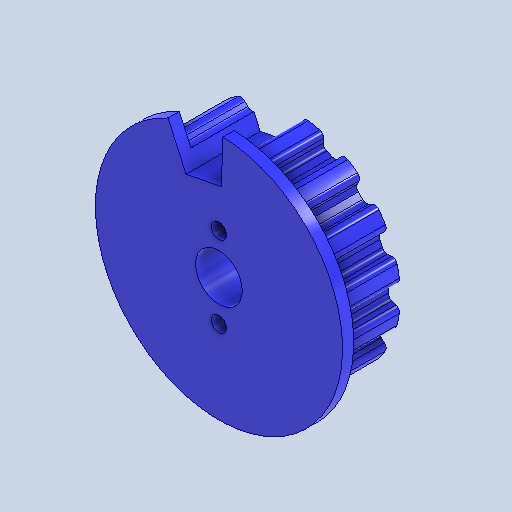
# Autodesk Inventor part: belt_liner_v2_3DP_P-1
Saved by Autodesk Inventor 2025.2 (Build 292293000, 293)
## iProperties
CustomPartVersion: 1
Created: 2024-12-08
Part Number: belt_liner_v2_3DP_P-1
Material: ABS プラスチック
Document SubType Name: Modeling
Designer: haruy
Density: 1.06 g/cm^3
Appearance: 青 - 壁塗料 - 光沢
Author: haruy
Autodesk Inventor part; units mm, degrees
ref_plane "YZ Plane" through (0, 0, 0) normal (1, 0, 0) x (0, 1, 0)
ref_plane "XZ Plane" through (0, 0, 0) normal (0, 1, 0) x (-1, 0, 0)
sketch "プーリ スケッチ" plane through (0, 0, 0) normal (0, 0, 1) x (1, 0, 0)
  circle A0 centre (0, 0) radius 24.2552 construction
  circle A1 centre (0, 0) radius 23.8742
  circle A2 centre (0, 0) radius 21.2072
  line L0 (-2.4489, 23.7483) -> (-1.524, 21.2072)
  line L1 (-1.524, 21.2072) -> (1.524, 21.2072)
  line L2 (1.524, 21.2072) -> (2.4489, 23.7483)
  line L3 (0, 0) -> (0, 23.8742) construction
  point P0 (0, 21.2072)
  dimension "d0" = 48.5104
  dimension "d1" = 0.381
  dimension "d2" = 2.667
  dimension "d3" = 40
  dimension "d4" = 3.048
  constraints: 8 end point, 3 coincident, 3 point on circle, 2 centre point, 1 horizontal, 1 midpoint, 1 point on line, 1 vertical, 1 vertical alignment, 3 other
  measures "d0" diameter of A0
  measures "d1" radial gap between concentric circles of A0 A1
  measures "d3" angle of L2 L0
  measures "d4" distance of L0.end L1.end
extrude "基本ボディ" add sketch "プーリ スケッチ" along normal mid plane 14 contours A2 | A1 L0 L1 L2 | L2 L1 L0 A1
extrude "歯" cut sketch "プーリ スケッチ" along normal through all both and the other way through all contours L2 L1 L0 A1 picked at (0, 22.9759)
fillet "Fillet" radius 1.1938 2 edges at (1.524, 21.2072, 0) (-1.524, 21.2072, 0)
fillet "Fillet" radius 1.1684 4 edges at (-2.4489, 23.7483, 3.5) (-2.4489, 23.7483, -3.5) (2.4489, 23.7483, 3.5) (2.4489, 23.7483, -3.5)
pattern_circular "Teeth" count 16 over 360 about axis through (0, 0, -10) along (0, 0, 1) of "歯", "Fillet"
sketch "スケッチ2" plane through (0, 0, 7) normal (0, 0, 1) x (1, 0, 0)
  circle A0 centre (0, 0) radius 27.5
  dimension "d17" = 55
  constraints: 1 centre point, 1 coincident
  measures "d17" diameter of A0
extrude "押し出し3" add sketch "スケッチ2" along normal blind 2.5
ref_plane "作業平面1" through (0, 0, 0) normal (0, 0, -1) x (-1, 0, 0)
mirror "ミラー1" [suppressed]
sketch "スケッチ3" plane through (0, 0, 9.5) normal (0, 0, 1) x (1, 0, 0)
  circle A0 centre (0, 0) radius 5.2
  circle A1 centre (0, 9) radius 1.7
  circle A2 centre (0, -9) radius 1.7
  dimension "d21" = 10.4
  dimension "d22" = 3.4
  dimension "d23" = 9
  dimension "d26" = 360
  constraints: 3 centre point, 1 coincident, 5 other
  measures "d21" diameter of A0
  measures "d22" diameter of A1
  measures "d23" distance of A1.centre point (0, 0)
extrude "押し出し4" cut sketch "スケッチ3" against normal through all
sketch "スケッチ4" plane through (0, 0, -7) normal (0, 0, -1) x (-1, 0, 0)
  line L0 (-35.8556, 31.439) -> (48.4071, 14.6781)
  arc A0 (5.9069, 23.132) -> (3.395, 23.6316) centre (0, 0) ccw projected
  line L1 (3.395, 23.6316) -> (5.9069, 23.132)
  line L2 (2.199, 23.8695) -> (1.6137, 20.9271)
  line L3 (0, 0) -> (4.6509, 23.3818)
  line L4 (2.6894, 23.772) -> (6.6125, 22.9916)
  line L5 (6.6125, 22.9916) -> (6.0272, 20.0492)
  line L6 (6.0272, 20.0492) -> (2.1041, 20.8296)
  line L7 (2.1041, 20.8296) -> (2.6894, 23.772)
  line L8 (2.199, 23.8695) -> (7.1029, 22.894)
  line L9 (7.1029, 22.894) -> (9.0538, 32.7019)
  line L10 (9.0538, 32.7019) -> (4.1499, 33.6773)
  line L11 (4.1499, 33.6773) -> (2.199, 23.8695)
  line L12 (8.6743, 20.5423) -> (11.4055, 34.2733)
  line L13 (11.4055, 34.2733) -> (2.5785, 36.0291)
  line L14 (2.5785, 36.0291) -> (-0.1528, 22.2981)
  line L15 (1.118, 26.1237) -> (8.9642, 24.563)
  line L16 (8.9642, 24.563) -> (7.5986, 17.6975)
  line L17 (7.5986, 17.6975) -> (-0.2477, 19.2582)
  line L18 (-0.2477, 19.2582) -> (1.118, 26.1237)
  line L19 (-0.1528, 22.2981) -> (-0.7381, 19.3558)
  line L20 (-0.7381, 19.3558) -> (-0.2477, 19.2582)
  line L21 (8.6743, 20.5423) -> (8.089, 17.5999)
  line L22 (8.089, 17.5999) -> (7.5986, 17.6975)
  line L23 (-11.4055, 34.2733) -> (-8.6743, 20.5423)
  line L24 (-8.6743, 20.5423) -> (-8.089, 17.5999)
  line L25 (0.2477, 19.2582) -> (-7.5986, 17.6975)
  line L26 (-8.089, 17.5999) -> (-7.5986, 17.6975)
  line L27 (0.7381, 19.3558) -> (0.2477, 19.2582)
  line L28 (0.1528, 22.2981) -> (0.7381, 19.3558)
  line L29 (0.1528, 22.2981) -> (-2.5785, 36.0291)
  line L30 (-23.6532, 27.2997) -> (-15.8752, 15.6591)
  line L31 (-15.8752, 15.6591) -> (-14.2085, 13.1647)
  line L32 (-7.141, 17.887) -> (-13.7927, 13.4425)
  line L33 (-14.2085, 13.1647) -> (-13.7927, 13.4425)
  line L34 (-6.7252, 18.1648) -> (-7.141, 17.887)
  line L35 (-8.392, 20.6592) -> (-6.7252, 18.1648)
  line L36 (-8.392, 20.6592) -> (-16.1699, 32.2998)
  line L37 (-32.2998, 16.1699) -> (-20.6592, 8.392)
  line L38 (-20.6592, 8.392) -> (-18.1648, 6.7252)
  line L39 (-13.4425, 13.7927) -> (-17.887, 7.141)
  line L40 (-18.1648, 6.7252) -> (-17.887, 7.141)
  line L41 (-13.1647, 14.2085) -> (-13.4425, 13.7927)
  line L42 (-15.6591, 15.8752) -> (-13.1647, 14.2085)
  line L43 (-15.6591, 15.8752) -> (-27.2997, 23.6532)
  line L44 (-36.0291, 2.5785) -> (-22.2981, -0.1528)
  line L45 (-22.2981, -0.1528) -> (-19.3558, -0.7381)
  line L46 (-17.6975, 7.5986) -> (-19.2582, -0.2477)
  line L47 (-19.3558, -0.7381) -> (-19.2582, -0.2477)
  line L48 (-17.5999, 8.089) -> (-17.6975, 7.5986)
  line L49 (-20.5423, 8.6743) -> (-17.5999, 8.089)
  line L50 (-20.5423, 8.6743) -> (-34.2733, 11.4055)
  line L51 (-34.2733, -11.4055) -> (-20.5423, -8.6743)
  line L52 (-20.5423, -8.6743) -> (-17.5999, -8.089)
  line L53 (-19.2582, 0.2477) -> (-17.6975, -7.5986)
  line L54 (-17.5999, -8.089) -> (-17.6975, -7.5986)
  line L55 (-19.3558, 0.7381) -> (-19.2582, 0.2477)
  line L56 (-22.2981, 0.1528) -> (-19.3558, 0.7381)
  line L57 (-22.2981, 0.1528) -> (-36.0291, -2.5785)
  line L58 (-27.2997, -23.6532) -> (-15.6591, -15.8752)
  line L59 (-15.6591, -15.8752) -> (-13.1647, -14.2085)
  line L60 (-17.887, -7.141) -> (-13.4425, -13.7927)
  line L61 (-13.1647, -14.2085) -> (-13.4425, -13.7927)
  line L62 (-18.1648, -6.7252) -> (-17.887, -7.141)
  line L63 (-20.6592, -8.392) -> (-18.1648, -6.7252)
  line L64 (-20.6592, -8.392) -> (-32.2998, -16.1699)
  line L65 (-16.1699, -32.2998) -> (-8.392, -20.6592)
  line L66 (-8.392, -20.6592) -> (-6.7252, -18.1648)
  line L67 (-13.7927, -13.4425) -> (-7.141, -17.887)
  line L68 (-6.7252, -18.1648) -> (-7.141, -17.887)
  line L69 (-14.2085, -13.1647) -> (-13.7927, -13.4425)
  line L70 (-15.8752, -15.6591) -> (-14.2085, -13.1647)
  line L71 (-15.8752, -15.6591) -> (-23.6532, -27.2997)
  line L72 (-2.5785, -36.0291) -> (0.1528, -22.2981)
  line L73 (0.1528, -22.2981) -> (0.7381, -19.3558)
  line L74 (-7.5986, -17.6975) -> (0.2477, -19.2582)
  line L75 (0.7381, -19.3558) -> (0.2477, -19.2582)
  line L76 (-8.089, -17.5999) -> (-7.5986, -17.6975)
  line L77 (-8.6743, -20.5423) -> (-8.089, -17.5999)
  line L78 (-8.6743, -20.5423) -> (-11.4055, -34.2733)
  line L79 (11.4055, -34.2733) -> (8.6743, -20.5423)
  line L80 (8.6743, -20.5423) -> (8.089, -17.5999)
  line L81 (-0.2477, -19.2582) -> (7.5986, -17.6975)
  line L82 (8.089, -17.5999) -> (7.5986, -17.6975)
  line L83 (-0.7381, -19.3558) -> (-0.2477, -19.2582)
  line L84 (-0.1528, -22.2981) -> (-0.7381, -19.3558)
  line L85 (-0.1528, -22.2981) -> (2.5785, -36.0291)
  line L86 (23.6532, -27.2997) -> (15.8752, -15.6591)
  line L87 (15.8752, -15.6591) -> (14.2085, -13.1647)
  line L88 (7.141, -17.887) -> (13.7927, -13.4425)
  line L89 (14.2085, -13.1647) -> (13.7927, -13.4425)
  line L90 (6.7252, -18.1648) -> (7.141, -17.887)
  line L91 (8.392, -20.6592) -> (6.7252, -18.1648)
  line L92 (8.392, -20.6592) -> (16.1699, -32.2998)
  line L93 (32.2998, -16.1699) -> (20.6592, -8.392)
  line L94 (20.6592, -8.392) -> (18.1648, -6.7252)
  line L95 (13.4425, -13.7927) -> (17.887, -7.141)
  line L96 (18.1648, -6.7252) -> (17.887, -7.141)
  line L97 (13.1647, -14.2085) -> (13.4425, -13.7927)
  line L98 (15.6591, -15.8752) -> (13.1647, -14.2085)
  line L99 (15.6591, -15.8752) -> (27.2997, -23.6532)
  line L100 (36.0291, -2.5785) -> (22.2981, 0.1528)
  line L101 (22.2981, 0.1528) -> (19.3558, 0.7381)
  line L102 (17.6975, -7.5986) -> (19.2582, 0.2477)
  line L103 (19.3558, 0.7381) -> (19.2582, 0.2477)
  line L104 (17.5999, -8.089) -> (17.6975, -7.5986)
  line L105 (20.5423, -8.6743) -> (17.5999, -8.089)
  line L106 (20.5423, -8.6743) -> (34.2733, -11.4055)
  line L107 (34.2733, 11.4055) -> (20.5423, 8.6743)
  line L108 (20.5423, 8.6743) -> (17.5999, 8.089)
  line L109 (19.2582, -0.2477) -> (17.6975, 7.5986)
  line L110 (17.5999, 8.089) -> (17.6975, 7.5986)
  line L111 (19.3558, -0.7381) -> (19.2582, -0.2477)
  line L112 (22.2981, -0.1528) -> (19.3558, -0.7381)
  line L113 (22.2981, -0.1528) -> (36.0291, 2.5785)
  line L114 (27.2997, 23.6532) -> (15.6591, 15.8752)
  line L115 (15.6591, 15.8752) -> (13.1647, 14.2085)
  line L116 (17.887, 7.141) -> (13.4425, 13.7927)
  line L117 (13.1647, 14.2085) -> (13.4425, 13.7927)
  line L118 (18.1648, 6.7252) -> (17.887, 7.141)
  line L119 (20.6592, 8.392) -> (18.1648, 6.7252)
  line L120 (20.6592, 8.392) -> (32.2998, 16.1699)
  line L121 (16.1699, 32.2998) -> (8.392, 20.6592)
  line L122 (8.392, 20.6592) -> (6.7252, 18.1648)
  line L123 (13.7927, 13.4425) -> (7.141, 17.887)
  line L124 (6.7252, 18.1648) -> (7.141, 17.887)
  line L125 (14.2085, 13.1647) -> (13.7927, 13.4425)
  line L126 (15.8752, 15.6591) -> (14.2085, 13.1647)
  line L127 (15.8752, 15.6591) -> (23.6532, 27.2997)
  line L128 (13.4918, 31.8191) -> (11.5409, 22.0113)
  line L129 (18.3958, 30.8437) -> (13.4918, 31.8191)
  line L130 (16.4449, 21.0358) -> (18.3958, 30.8437)
  line L131 (11.5409, 22.0113) -> (16.4449, 21.0358)
  line L132 (11.4461, 18.9714) -> (12.0313, 21.9137)
  line L133 (15.3692, 18.191) -> (11.4461, 18.9714)
  line L134 (15.9545, 21.1334) -> (15.3692, 18.191)
  line L135 (22.8338, 29.9609) -> (20.8829, 20.153)
  line L136 (27.7377, 28.9854) -> (22.8338, 29.9609)
  line L137 (25.7868, 19.1776) -> (27.7377, 28.9854)
  line L138 (20.8829, 20.153) -> (25.7868, 19.1776)
  line L139 (20.788, 17.1131) -> (21.3733, 20.0555)
  line L140 (24.7112, 16.3328) -> (20.788, 17.1131)
  line L141 (25.2965, 19.2751) -> (24.7112, 16.3328)
  circle A1 centre (0, 0) radius 27.5
  line L142 (-0.8791, 27.4859) -> (0.7989, 19.05)
  line L143 (11.3306, 25.0573) -> (6.5521, 17.9057)
  line L144 (0.1425, 21.2198) -> (7.9888, 19.6591)
  line L145 (7.9888, 19.6591) -> (7.306, 16.2263)
  line L146 (7.306, 16.2263) -> (-0.5403, 17.787)
  line L147 (-0.5403, 17.787) -> (0.1425, 21.2198)
  line L148 (-0.5403, 17.787) -> (-0.8791, 27.4859)
  line L149 (7.306, 16.2263) -> (11.3306, 25.0573)
  point P0 (4.6576, 23.4155)
  point P1 (0.7187, 19.4532)
  point P2 (7.2808, 18.9963)
  point P3 (11.3306, 25.0573)
  point P4 (11.3306, 25.0573)
  point P5 (7.4069, 17.7356)
  point P6 (-0.056, 19.2201)
  point P7 (0.543, 20.3365)
  point P8 (8.1012, 20.2241)
  point P9 (7.3509, 17.7467)
  point P10 (7.8477, 17.4149)
  point P11 (0.2549, 21.7848)
  point P12 (0, 19.2089)
  point P13 (-0.5859, 19.0924)
  point P14 (8.1012, 20.2241)
  point P15 (0.2549, 21.7848)
  dimension "d59" = 55
  dimension "d30" = 0
  dimension "d31" = 2.5
  dimension "d32" = 3
  dimension "d35" = 3
  dimension "d36" = 4
  dimension "d37" = 2
  dimension "d38" = 10
  dimension "d39" = 5
  dimension "d40" = 2.5
  dimension "d41" = 2
  dimension "d42" = 2
  dimension "d45" = 360
  dimension "d49" = 9.525
  dimension "d56" = 3.5
  dimension "d58" = 4
  dimension "d60" = 0
  dimension "d61" = 4
  constraints: 300 end point, 10 parallel, 7 point on line, 5 perpendicular, 3 collinear, 3 symmetric about line, 2 point on circle, 1 coincident, 1 midpoint, 280 other
  measures "d30" distance between parallel lines of L1 L0
  measures "d31" distance from line of L2 point (4.658, 23.415)
  measures "d32" distance from line of L0 L2.end
  measures "d35" distance between parallel lines of L0 L6
  measures "d36" distance between parallel lines of L5 L7
  measures "d37" distance between parallel lines of L3 L7
  measures "d38" distance between parallel lines of L8 L10
  measures "d39" distance between parallel lines of L9 L11
  measures "d40" distance between parallel lines of L3 L11
  measures "d41" distance between parallel lines of L11 L14
  measures "d42" distance between parallel lines of L7 L18
  measures "d49" distance of L10.end L128.start
  measures "d56" distance of L144.end L145.end
  measures "d58" distance between parallel lines of L3 L147
  measures "d60" distance between parallel lines of L6 L144
  measures "d61" distance between parallel lines of L3 L145
extrude "押し出し5" cut sketch "スケッチ4" along normal through all both and the other way through all contours L11 L15 L9 L0 A0 | L2 L144 L28 L18 L0 | L0 L7 L144 L2 | L0 L18 L15 L11 | L0 L3 L6 L7 | L18 L28 L29 L14 L0 | L0 L14 A1 L11 L15 L18 | L144 L6 L3 L17 L142 L28 | L11 A1 L9 L15 | A0 L0 | L14 L29 L0 | L0 L29 A1 L14 | L28 L144 L18 | L18 L20 L148 L19 L14 L29 L28 | L28 L27 L25 L17 L18 L144 | L15 L16 L0 L9 | L9 A1 L12 L0 L16 L15 | L0 L5 L6 L3 | L6 L144 L122 L143 L17 L3 | L29 L14 L19 L148 L0 | L0 L148 L29 | L142 L17 L25 L27 | L0 L16 L122 L144 L5 | L17 L123 L145 L146 L3 | L3 L146 L147 L25 L17 | L147 L25 L148 L20 | L17 L25 L147 | A1 L121 L0 L12 | L0 L12 L121 L122 L16 | L143 L124 L123 L17 | L144 L16 L17 L123 L124 L122 | L122 L16 L144 | L147 L148 L25 | L0 L121 L12 | L149 L0 L121 | L122 L121 L12 L21 L149 L22 L16 | L145 L123 L149 | L17 L145 L123 | L0 L149 L21 L12 L121 | L145 L22 L149 L123
sketch "スケッチ5" plane through (0, 0, 9.5) normal (0, 0, 1) x (1, 0, 0)
  arc A0 (-11.3306, 25.0573) -> (0.8791, 27.4859) centre (0, 0) ccw projected
  circle A1 centre (0, -9) radius 1.7 projected
  circle A2 centre (0, 9) radius 1.7 projected
  circle A3 centre (0, 0) radius 5.2 projected
  line L0 (-7.306, 16.2263) -> (-11.3306, 25.0573) projected
  line L1 (0.8791, 27.4859) -> (0.5403, 17.787) projected
  line L2 (0.5403, 17.787) -> (-7.306, 16.2263) projected
equation "\"d1\" = da_a"
equation "\"d2\" = da_hg"
equation "\"d3\" = 2 * da_fi"
equation "\"d4\" = da_bw"
equation "\"d5\" = da_bf"
equation "\"d7\" = da_bf"
equation "\"d9\" = da_rb"
equation "\"d10\" = da_rt"
equation "\"da_pb\" = 9.525"
equation "\"da_fi\" = 20deg"
equation "\"da_hg\" = 2.667"
equation "\"da_bw\" = 3.048"
equation "\"da_rb\" = 1.1938"
equation "\"da_rt\" = 1.1684"
equation "\"da_a\" = 0.381"
equation "\"da_bf\" = 14"
equation "\"da_wf\" = 1.27"
equation "\"da_hf\" = 1.651"
body "Solid1"
